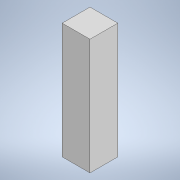
# Autodesk Inventor part: Attachment_Shaft
Saved by Autodesk Inventor 2022 (Build 260153000, 153)
## iProperties
Created: 2022-01-03
Part Number: Attachment_Shaft
Material: Generic
Document SubType Name: Modeling
Designer: Mlees
Density: 1 g/cm^3
Appearance: Default
Author: Mlees
Autodesk Inventor part; units mm, degrees
ref_plane "YZ Plane" through (0, 0, 0) normal (1, 0, 0) x (0, 1, 0)
ref_plane "XZ Plane" through (0, 0, 0) normal (0, 1, 0) x (-1, 0, 0)
ref_plane "XY Plane" through (0, 0, 0) normal (0, 0, 1) x (1, 0, 0)
sketch "Sketch1" plane through (0, 0, 0) normal (0, 1, 0) x (-1, 0, 0)
  line L0 (0, 0) -> (24.4, 0)
  line L1 (24.4, 0) -> (24.4, -24.4)
  line L2 (24.4, -24.4) -> (0, -24.4)
  line L3 (0, -24.4) -> (0, 0)
  dimension "d0" = 24.4
  dimension "d1" = 24.4
  constraints: 8 end point, 2 parallel, 1 horizontal, 1 perpendicular
  measures "d0" distance of L1.end L2.end
  measures "d1" distance of L0.end L1.end
extrude "Extrusion1" add sketch "Sketch1" along normal blind 101.6
body "Solid1"
